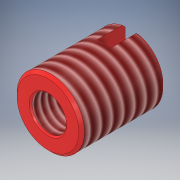
# Autodesk Inventor part: XGEN_M3_draadbus_4x6mm
Saved by Autodesk Inventor 2019 (Build 230136000, 136)
## iProperties
Created: 2019-03-01
Part Number: XGEN_M3_draadbus_4x6mm
Material: Generic
Document SubType Name: Modeling
Designer: Rene
Density: 1 g/cm^3
Appearance: Light Red
Author: Rene
Autodesk Inventor part; units mm, degrees
ref_plane "YZ Plane" through (0, 0, 0) normal (1, 0, 0) x (0, 1, 0)
ref_plane "XZ Plane" through (0, 0, 0) normal (0, 1, 0) x (-1, 0, 0)
ref_plane "XY Plane" through (0, 0, 0) normal (0, 0, 1) x (1, 0, 0)
sketch "Sketch1" plane through (0, 0, 0) normal (0, 0, 1) x (1, 0, 0)
  circle A0 centre (0, 0) radius 2.4
  dimension "d0" = 4.8
  constraints: 1 centre point, 1 coincident
  measures "d0" diameter of A0
extrude "Extrusion1" add sketch "Sketch1" along normal blind 6
sketch "Sketch2" plane through (0, 0, 6) normal (0, 0, 1) x (1, 0, 0)
  point P0 (0, 0)
  point P1 (0, 0)
  constraints: 1 coincident
hole "Hole1" at (0, 0, 6) direction (0, 0, -1) diameter 2.459 end through all thread size "M3x0.5" class "6H" standard "ISO Metric profile"
chamfer "Chamfer1" distance 0.2 angle 45 2 edges at (-2.4, 0, 6) (-2.4, 0, 0)
chamfer "Chamfer2" distance 0.1 angle 45 2 edges at (0, 1.2295, 6) (0, 1.2295, 0)
thread "Thread2" size "M5x0.8" class "6g" standard "ANSI Metric M Profile" full length
sketch "Sketch4" plane through (0, 0, 0) normal (0, 1, 0) x (-1, 0, 0)
  line L0 (-0.5, 0) -> (0.5, 0)
  line L1 (0.5, 0) -> (0.5, 2)
  line L2 (0.5, 2) -> (-0.5, 2)
  line L3 (-0.5, 2) -> (-0.5, 0)
  point P0 (0, 0)
  dimension "d22" = 1
  dimension "d23" = 0.5
  dimension "d24" = 2
  constraints: 8 end point, 2 parallel, 1 horizontal, 1 perpendicular
  measures "d22" distance of L0.end L0.start
  measures "d23" distance of point (0, 0) L0.start
  measures "d24" distance of L2.end L0.start
extrude "Extrusion2" cut sketch "Sketch4" along normal mid plane 6
equation "\"d23\" = 0.5 * d22"
body "Solid1"
